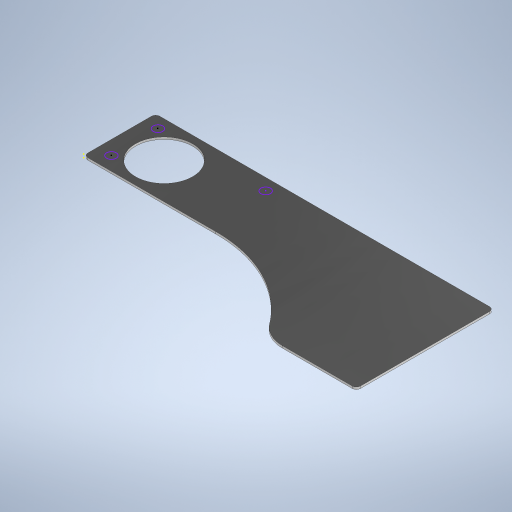
# Autodesk Inventor part: chapa_carbono_lateral_oposto
Saved by Autodesk Inventor 2024 (Build 280153000, 153)
## iProperties
Created: 2024-10-14
Part Number: chapa_carbono_lateral_oposto
Material: Genérico
Document SubType Name: Modeling
Designer: robof
Density: 1 g/cm^3
Appearance: Padrão
Author: robof
Autodesk Inventor part; units mm, degrees
ref_plane "YZ Plane" through (0, 0, 0) normal (1, 0, 0) x (0, 1, 0)
ref_plane "XZ Plane" through (0, 0, 0) normal (0, 1, 0) x (-1, 0, 0)
ref_plane "XY Plane" through (0, 0, 0) normal (0, 0, 1) x (1, 0, 0)
sketch "Esboço1" plane through (0, 0, 0) normal (0, 1, 0) x (-1, 0, 0)
  line L0 (0, 0) -> (-160, 0)
  line L1 (-160, 0) -> (-160, -34)
  line L2 (-160, -34) -> (0, -34)
  line L3 (0, -34) -> (0, 0)
  line L4 (0, 0) -> (-4, 0)
  line L5 (-4, 0) -> (-62.5, 0)
  line L6 (-160, -34) -> (-160, 31)
  line L7 (-160, -34) -> (-117, -34)
  line L8 (-117, -34) -> (-117, 31)
  line L9 (-117, 31) -> (-160, 31)
  line L10 (-160, 31) -> (-160, -34)
  arc A0 (-117, 31) -> (-62.5, 0) centre (-62.5, 63.4073) ccw
  dimension "d0" = 160
  dimension "d1" = 34
  dimension "d2" = 4
  dimension "d3" = 58.5
  dimension "d4" = 65
  dimension "d5" = 43
  constraints: 22 end point, 4 parallel, 3 point on line, 2 horizontal, 2 perpendicular, 2 point on circle, 1 centre point, 1 tangent
  measures "d0" distance of L2.end L1.end
  measures "d1" distance of L1.end L0.end
  measures "d2" distance of L0.start L4.end
  measures "d3" distance of L4.end L5.end
  measures "d4" distance of L1.end L6.end
  measures "d5" distance of L9.end L8.end
extrude "Extrusão1" add sketch "Esboço1" along normal blind 1
fillet "Arredondamento1" radius 2 4 edges at (160, 0.5, 31) (160, 0.5, -34) (0, 0.5, 0) (0, 0.5, -34)
fillet "Arredondamento2" radius 15 1 edges at (117, 0.5, 31)
sketch "Esboço5" plane through (0, 1, 0) normal (0, 1, 0) x (1, 0, 0)
  line L0 (160, -29) -> (160, 32) projected
  line L1 (160, -21.1735) -> (160, -7.1735)
  line L2 (160, -21.1735) -> (146, -21.1735)
  line L3 (124.952, -31) -> (158, -31) projected
  line L4 (146, -31) -> (139, -31)
  line L5 (146, -31) -> (146, -24)
  circle A0 centre (146, -24) radius 3.5
  line L6 (146, -24) -> (130, -24)
  circle A1 centre (130, -24) radius 3.5
  line L7 (146, -24) -> (146, 8)
  circle A2 centre (146, 8) radius 3.5
  line L8 (146, 8) -> (130, 8)
  circle A3 centre (130, 8) radius 3.5
  point P0 (0, 0)
  dimension "d32" = 14
  dimension "d33" = 14
  dimension "d34" = 7
  dimension "d35" = 7
  dimension "d36" = 7
  dimension "d37" = 16
  dimension "d38" = 7
  dimension "d39" = 32
  dimension "d40" = 7
  dimension "d41" = 7
  constraints: 14 end point, 4 centre point, 4 coincident, 4 point on line, 3 horizontal, 2 vertical
  measures "d32" distance of L1.start L1.end
  measures "d33" distance of L1.start L2.end
  measures "d34" distance of L4.start L4.end
  measures "d35" distance of L4.start L5.end
  measures "d36" diameter of A0
  measures "d37" distance of L6.start L6.end
  measures "d38" diameter of A1
  measures "d39" distance of L6.start L7.end
  measures "d40" diameter of A2
  measures "d41" diameter of A3
extrude "Extrusão3" add sketch "Esboço5" along normal blind 1
sketch "Esboço6" plane through (130, 2, -8) normal (0, 1, 0) x (1, 0, 0)
  circle A0 centre (0, 0) radius 2.25
  circle A1 centre (16, 0) radius 3.5 projected
  circle A2 centre (16, 0) radius 2.25
  circle A3 centre (0, -32) radius 3.5 projected
  circle A4 centre (0, -32) radius 2.25
  circle A5 centre (16, -32) radius 3.5 projected
  circle A6 centre (16, -32) radius 2.25
  point P0 (-130, -8)
  dimension "d44" = 4.5
  dimension "d45" = 4.5
  dimension "d46" = 4.5
  dimension "d47" = 4.5
  constraints: 4 centre point, 3 coincident
  measures "d44" diameter of A0
  measures "d45" diameter of A2
  measures "d46" diameter of A4
  measures "d47" diameter of A6
extrude "Extrusão4" add sketch "Esboço6" along normal blind 2.5 contours A0 | A2 | A4 | A6
sketch "Esboço7" plane through (130, 4.5, -8) normal (0, 1, 0) x (1, 0, 0)
  circle A0 centre (0, 0) radius 2.25 projected
  line L0 (-0.7066, -1.2286) -> (-1.4173, -0.0023)
  line L1 (-1.4173, -0.0023) -> (-0.7107, 1.2262)
  line L2 (-0.7107, 1.2262) -> (0.7066, 1.2286)
  line L3 (0.7066, 1.2286) -> (1.4173, 0.0023)
  line L4 (1.4173, 0.0023) -> (0.7107, -1.2262)
  line L5 (0.7107, -1.2262) -> (-0.7066, -1.2286)
  line L6 (0, 0) -> (8, 0)
  line L7 (8, 0) -> (8, -3.5397)
  circle A1 centre (16, 0) radius 2.25
  line L8 (16.7066, -1.2286) -> (17.4173, -0.0023)
  line L9 (17.4173, -0.0023) -> (16.7107, 1.2262)
  line L10 (16.7107, 1.2262) -> (15.2934, 1.2286)
  line L11 (15.2934, 1.2286) -> (14.5827, 0.0023)
  line L12 (14.5827, 0.0023) -> (15.2893, -1.2262)
  line L13 (15.2893, -1.2262) -> (16.7066, -1.2286)
  line L14 (0, 0) -> (0, -16)
  line L15 (0, -16) -> (6.7888, -16)
  circle A2 centre (0, -32) radius 2.25
  line L16 (-0.7066, -30.7714) -> (-1.4173, -31.9977)
  line L17 (-1.4173, -31.9977) -> (-0.7107, -33.2262)
  line L18 (-0.7107, -33.2262) -> (0.7066, -33.2286)
  line L19 (0.7066, -33.2286) -> (1.4173, -32.0023)
  line L20 (1.4173, -32.0023) -> (0.7107, -30.7738)
  line L21 (0.7107, -30.7738) -> (-0.7066, -30.7714)
  circle A3 centre (16, -32) radius 2.25
  line L22 (16.7066, -30.7714) -> (17.4173, -31.9977)
  line L23 (17.4173, -31.9977) -> (16.7107, -33.2262)
  line L24 (16.7107, -33.2262) -> (15.2934, -33.2286)
  line L25 (15.2934, -33.2286) -> (14.5827, -32.0023)
  line L26 (14.5827, -32.0023) -> (15.2893, -30.7738)
  line L27 (15.2893, -30.7738) -> (16.7066, -30.7714)
  point P0 (-130, -8)
  dimension "d50" = 8
  dimension "d51" = 16
  constraints: 56 end point, 24 symmetric about line, 4 coincident, 3 centre point, 2 perpendicular, 1 horizontal, 1 vertical, 16 other
  measures "d50" distance of L6.start L6.end
  measures "d51" distance of L6.start L14.end
extrude "Extrusão5" cut sketch "Esboço7" against normal blind 1.5 contours L6 L14 L5 L0 L1 L2 L3 L4 | L4 L5 L14 L6 | L13 L12 L11 L10 L9 L8 | L21 L20 L19 L18 L17 L16 | L22 L23 L24 L25 L26 L27
sketch "Esboço8" plane through (0, 1, 0) normal (0, 1, 0) x (1, 0, 0)
  line L0 (0, 0) -> (6, 0)
  line L1 (2, 0) -> (62.5, 0) projected
  line L2 (6, 0) -> (-1.5, 0)
  line L3 (6, 0) -> (6, 7.5)
  circle A0 centre (6, 7.5) radius 2.25
  line L4 (0, 32) -> (0, 2) projected
  line L5 (0, 17) -> (13.7618, 17)
  circle A1 centre (6, 26.5) radius 2.25
  dimension "d54" = 6
  dimension "d55" = 7.5
  dimension "d56" = 7.5
  dimension "d57" = 4.5
  constraints: 8 end point, 2 centre point, 2 point on line, 1 coincident, 1 horizontal, 1 midpoint, 1 symmetric about line, 1 vertical, 1 other
  measures "d54" distance of L0.start L0.end
  measures "d55" distance of L0.end L2.end
  measures "d56" distance of L0.end L3.end
  measures "d57" diameter of A0
extrude "Extrusão6" cut sketch "Esboço8" against normal blind 0.1
sketch "Esboço9" plane through (6, 0.9, -26.5) normal (0, 1, 0) x (1, 0, 0)
  circle A0 centre (0, -19) radius 2.25 projected
  line L0 (0, -19) -> (0.25, -19)
  line L1 (0.25, -19) -> (0.25, -20.5)
  line L2 (0.25, -20.5) -> (0, -20.5)
  line L3 (0, -20.5) -> (0, -19)
  line L4 (0, -20.5) -> (-0.25, -20.5)
  line L5 (-0.25, -20.5) -> (-0.25, -19)
  line L6 (-0.25, -19) -> (0, -19)
  line L7 (0, -19) -> (0, -20.5)
  line L8 (0.25, -20.5) -> (-0.25, -20.5)
  line L9 (-0.25, -20.5) -> (-0.25, -17.5)
  line L10 (-0.25, -17.5) -> (0.25, -17.5)
  line L11 (0.25, -17.5) -> (0.25, -20.5)
  line L12 (0, -19) -> (1.5, -19)
  line L13 (1.5, -19) -> (1.5, -18.75)
  line L14 (1.5, -18.75) -> (0, -18.75)
  line L15 (0, -18.75) -> (0, -19)
  line L16 (1.5, -18.75) -> (-1.5, -18.75)
  line L17 (-1.5, -18.75) -> (-1.5, -19.25)
  line L18 (-1.5, -19.25) -> (1.5, -19.25)
  line L19 (1.5, -19.25) -> (1.5, -18.75)
  line L20 (-6, 5.5) -> (-6, -24.5) projected
  line L21 (-6, -9.5) -> (4.7143, -9.5)
  line L22 (0, 0) -> (0.25, 0)
  line L23 (0.25, 0) -> (0.25, 1.5)
  line L24 (0.25, 1.5) -> (0, 1.5)
  line L25 (0, 1.5) -> (0, 0)
  line L26 (0, 1.5) -> (-0.25, 1.5)
  line L27 (-0.25, 1.5) -> (-0.25, 0)
  line L28 (-0.25, 0) -> (0, 0)
  line L29 (0, 0) -> (0, 1.5)
  line L30 (0.25, 1.5) -> (-0.25, 1.5)
  line L31 (-0.25, 1.5) -> (-0.25, -1.5)
  line L32 (-0.25, -1.5) -> (0.25, -1.5)
  line L33 (0.25, -1.5) -> (0.25, 1.5)
  line L34 (0, 0) -> (1.5, 0)
  line L35 (1.5, 0) -> (1.5, -0.25)
  line L36 (1.5, -0.25) -> (0, -0.25)
  line L37 (0, -0.25) -> (0, 0)
  line L38 (1.5, -0.25) -> (-1.5, -0.25)
  line L39 (-1.5, -0.25) -> (-1.5, 0.25)
  line L40 (-1.5, 0.25) -> (1.5, 0.25)
  line L41 (1.5, 0.25) -> (1.5, -0.25)
  point P0 (-6, -26.5)
  point P1 (-0.25, -19.25)
  point P2 (0.25, -19.25)
  point P3 (0.25, -18.75)
  point P4 (-0.25, -18.75)
  point P5 (0.25, 0.25)
  point P6 (-0.25, 0.25)
  point P7 (-0.25, -0.25)
  point P8 (0.25, -0.25)
  dimension "d60" = 0.25
  dimension "d61" = 1.5
  dimension "d62" = 0.25
  dimension "d63" = 3
  dimension "d64" = 1.5
  dimension "d65" = 0.25
  dimension "d66" = 3
  dimension "d67" = 0.5
  constraints: 82 end point, 16 symmetric about line, 10 parallel, 6 horizontal, 5 perpendicular, 4 point on line, 1 midpoint
  measures "d60" distance of L1.end L2.end
  measures "d61" distance of L0.end L1.end
  measures "d62" distance of L5.end L6.end
  measures "d63" distance of L8.end L9.end
  measures "d64" distance of L14.end L13.end
  measures "d65" distance of L13.end L12.end
  measures "d66" distance of L18.end L17.end
  measures "d67" distance of L17.end L16.end
extrude "Extrusão7" cut sketch "Esboço9" against normal blind 0.1 contours L15 L14 L11 L0 | L0 L1 L18 L3 | L3 L18 L5 L6 | L6 L9 L16 L15 | L12 L19 L18 L1 | L11 L14 L13 L12 | L18 L1 L2 L3 | L3 L4 L5 L18 | L5 L18 L17 L16 L9 | L16 L9 L10 L11 L14 | L25 L40 L23 L22 | L28 L27 L40 L25 | L37 L38 L31 L28 | L22 L33 L36 L37 | L34 L35 L36 L33 | L23 L40 L41 L34 | L40 L27 L26 L25 | L25 L24 L23 L40 | L31 L38 L39 L40 L27 | L36 L33 L32 L31 L38
sketch "Esboço10" plane through (6, 0.9, -26.5) normal (0, 1, 0) x (1, 0, 0)
  line L0 (0, 0) -> (52, 0)
  circle A0 centre (52, 0) radius 2.25
  circle A1 centre (0, -19) radius 2.25 projected
  line L1 (0, -19) -> (52, -19)
  circle A2 centre (52, -19) radius 2.25
  point P0 (-6, -26.5)
  dimension "d70" = 52
  dimension "d71" = 4.5
  dimension "d72" = 52
  dimension "d73" = 4.5
  constraints: 4 end point, 2 centre point, 2 coincident, 1 horizontal, 1 parallel
  measures "d70" distance of L0.start L0.end
  measures "d71" diameter of A0
  measures "d72" distance of L1.start L1.end
  measures "d73" diameter of A2
extrude "Extrusão8" cut sketch "Esboço10" along normal blind 2 contours A0 | A2
sketch "Esboço11" plane through (58, 0.9, -26.5) normal (0, 1, 0) x (1, 0, 0)
  line L0 (0, 0) -> (0.25, 0)
  line L1 (0.25, 0) -> (0.25, 1.5)
  line L2 (0.25, 1.5) -> (0, 1.5)
  line L3 (0, 1.5) -> (0, 0)
  line L4 (0.25, 1.5) -> (-0.25, 1.5)
  line L5 (-0.25, 1.5) -> (-0.25, -1.5)
  line L6 (-0.25, -1.5) -> (0.25, -1.5)
  line L7 (0.25, -1.5) -> (0.25, 1.5)
  line L8 (0, 0) -> (1.5, 0)
  line L9 (1.5, 0) -> (1.5, 0.25)
  line L10 (1.5, 0.25) -> (0, 0.25)
  line L11 (0, 0.25) -> (0, 0)
  line L12 (1.5, 0.25) -> (-1.5, 0.25)
  line L13 (-1.5, 0.25) -> (-1.5, -0.25)
  line L14 (-1.5, -0.25) -> (1.5, -0.25)
  line L15 (1.5, -0.25) -> (1.5, 0.25)
  line L16 (-58, 5.5) -> (-58, -24.5) projected
  line L17 (-58, -9.5) -> (-46.2393, -9.5)
  line L18 (0, -19) -> (0.25, -19)
  line L19 (0.25, -19) -> (0.25, -20.5)
  line L20 (0.25, -20.5) -> (0, -20.5)
  line L21 (0, -20.5) -> (0, -19)
  line L22 (0.25, -20.5) -> (-0.25, -20.5)
  line L23 (-0.25, -20.5) -> (-0.25, -17.5)
  line L24 (-0.25, -17.5) -> (0.25, -17.5)
  line L25 (0.25, -17.5) -> (0.25, -20.5)
  line L26 (0, -19) -> (1.5, -19)
  line L27 (1.5, -19) -> (1.5, -19.25)
  line L28 (1.5, -19.25) -> (0, -19.25)
  line L29 (0, -19.25) -> (0, -19)
  line L30 (1.5, -19.25) -> (-1.5, -19.25)
  line L31 (-1.5, -19.25) -> (-1.5, -18.75)
  line L32 (-1.5, -18.75) -> (1.5, -18.75)
  line L33 (1.5, -18.75) -> (1.5, -19.25)
  point P0 (-58, -26.5)
  point P1 (0.25, -0.25)
  point P2 (1.5, 0)
  point P3 (0.25, 0.25)
  point P4 (0, 1.5)
  point P5 (-0.25, 0.25)
  point P6 (-0.25, -0.25)
  point P7 (0.25, -19.25)
  point P8 (1.5, -19)
  point P9 (0.25, -18.75)
  point P10 (-0.25, -18.75)
  point P11 (-0.25, -19.25)
  dimension "d76" = 0.25
  dimension "d77" = 1.5
  dimension "d78" = 0.5
  dimension "d79" = 3
  dimension "d80" = 1.5
  dimension "d81" = 0.25
  dimension "d82" = 3
  dimension "d83" = 0.5
  constraints: 66 end point, 13 symmetric about line, 8 parallel, 5 horizontal, 4 perpendicular, 1 midpoint
  measures "d76" distance of L2.end L1.end
  measures "d77" distance of L1.end L0.end
  measures "d78" distance of L6.end L5.end
  measures "d79" distance of L5.end L4.end
  measures "d80" distance of L10.end L9.end
  measures "d81" distance of L9.end L8.end
  measures "d82" distance of L14.end L13.end
  measures "d83" distance of L13.end L12.end
extrude "Extrusão9" cut sketch "Esboço11" against normal blind 0.1
sketch "Esboço12" plane through (0, 1, 0) normal (0, 1, 0) x (1, 0, 0)
  line L0 (0, 32) -> (0, 2) projected
  line L1 (0, 17) -> (5, 17)
  line L2 (5, 17) -> (36, 17)
  line L3 (5, 17) -> (20.5, 17)
  circle A0 centre (20.5, 17) radius 13
  point P0 (0, 0)
  dimension "d86" = 5
  dimension "d87" = 31
  dimension "d88" = 15.5
  dimension "d89" = 26
  constraints: 6 end point, 2 midpoint, 1 centre point, 1 coincident, 1 horizontal, 1 point on line
  measures "d86" distance of L1.start L1.end
  measures "d87" distance of L1.end L2.end
  measures "d88" distance of L1.end L3.end
  measures "d89" diameter of A0
extrude "Extrusão10" cut sketch "Esboço12" against normal blind 10
sketch "Esboço13" plane through (0, 1, 0) normal (0, 1, 0) x (1, 0, 0)
  circle A0 centre (20.5, 17) radius 13 projected
  circle A1 centre (20.5, 17) radius 13
  point P0 (0, 0)
  constraints: 1 centre point, 1 coincident
extrude "Extrusão11" add sketch "Esboço13" against normal blind 1
sketch "Esboço14" plane through (0, 1, 0) normal (0, 1, 0) x (1, 0, 0)
  line L0 (0, 32) -> (0, 2) projected
  line L1 (0, 17) -> (4.15, 17)
  line L2 (4.15, 17) -> (15.55, 17)
  line L3 (16.6408, 0) -> (16.6408, 6)
  circle A0 centre (15.55, 17) radius 11.054
  circle A1 centre (6, 7.5) radius 2.25 projected
  circle A2 centre (6, 7.5) radius 2.25
  circle A3 centre (6, 26.5) radius 2.25 projected
  circle A4 centre (6, 26.5) radius 2.25
  point P0 (0, 0)
  dimension "d94" = 4.15
  dimension "d95" = 11.4
  dimension "d97" = 6
  constraints: 6 end point, 3 coincident, 2 centre point, 2 horizontal, 1 midpoint, 1 vertical, 3 other
  measures "d94" distance of L1.start L1.end
  measures "d95" distance of L1.end L2.end
  measures "d97" distance of L3.start L3.end
extrude "Extrusão12" add sketch "Esboço14" against normal blind 1 contours A1 | A3
sketch "Esboço15" plane through (0, 1, 0) normal (0, 1, 0) x (1, 0, 0)
  circle A0 centre (58, 7.5) radius 2.25 projected
  circle A1 centre (58, 7.5) radius 2.25
  circle A2 centre (58, 26.5) radius 2.25 projected
  circle A3 centre (58, 26.5) radius 2.25
  point P0 (0, 0)
  constraints: 2 centre point, 2 coincident
extrude "Extrusão13" add sketch "Esboço15" against normal blind 1
sketch "Esboço16" plane through (0, 1, 0) normal (0, 1, 0) x (1, 0, 0)
  line L0 (0, 0) -> (7, 0)
  line L1 (7, 0) -> (7, 6)
  line L2 (7, 6) -> (0, 6)
  line L3 (0, 6) -> (0, 0)
  circle A0 centre (7, 6) radius 2.25
  line L4 (0, 32) -> (0, 2) projected
  line L5 (0, 17) -> (5.9961, 17)
  line L6 (7, 0) -> (32.5, 0)
  line L7 (2, 0) -> (62.5, 0) projected
  line L8 (32.5, 0) -> (32.5, 15.1049)
  circle A1 centre (7, 28) radius 2.25
  circle A2 centre (58, 6) radius 2.25
  circle A3 centre (58, 28) radius 2.25
  dimension "d102" = 7
  dimension "d103" = 6
  dimension "d104" = 4.5
  dimension "d105" = 25.5
  constraints: 14 end point, 4 centre point, 3 symmetric about line, 2 horizontal, 2 parallel, 1 coincident, 1 midpoint, 1 perpendicular, 1 point on line, 1 vertical, 3 other
  measures "d102" distance of L2.end L1.end
  measures "d103" distance of L1.end L0.end
  measures "d104" diameter of A0
  measures "d105" distance of L0.end L6.end
extrude "Extrusão14" cut sketch "Esboço16" against normal blind 1 contours A0 L2 L1 | L1 L2 A0 | A1 | A2 | A3
sketch "Esboço17" plane through (0, 1, 0) normal (0, 1, 0) x (1, 0, 0)
  line L0 (0, 32) -> (0, 2) projected
  line L1 (0, 17) -> (17, 17)
  line L2 (17, 17) -> (21, 17)
  circle A0 centre (21, 17) radius 13.5
  point P0 (0, 0)
  dimension "d108" = 17
  dimension "d109" = 4
  dimension "d110" = 27
  constraints: 4 end point, 2 horizontal, 1 centre point, 1 coincident, 1 midpoint
  measures "d108" distance of L1.start L1.end
  measures "d109" distance of L1.end L2.end
  measures "d110" diameter of A0
extrude "Extrusão15" cut sketch "Esboço17" against normal blind 1
sketch "Esboço18" plane through (0, 0, 0) normal (0, -1, 0) x (1, 0, 0)
  circle A0 centre (58, -6) radius 2.25 projected
  circle A1 centre (58, -6) radius 2.25
  circle A2 centre (58, -28) radius 2.25 projected
  circle A3 centre (58, -28) radius 2.25
  circle A4 centre (7, -28) radius 2.25 projected
  circle A5 centre (7, -28) radius 2.25
  circle A6 centre (7, -6) radius 2.25 projected
  circle A7 centre (7, -6) radius 2.25
  point P0 (0, 0)
  constraints: 4 centre point, 4 coincident
extrude "Extrusão16" add sketch "Esboço18" against normal blind 2
sketch "Esboço19" plane through (7, 2, -28) normal (0, 1, 0) x (1, 0, 0)
  circle A0 centre (0, 0) radius 2.25
  circle A1 centre (0, -22) radius 2.25 projected
  circle A2 centre (0, -22) radius 2.25
  circle A3 centre (51, 0) radius 2.25 projected
  circle A4 centre (51, 0) radius 2.25
  circle A5 centre (51, -22) radius 2.25 projected
  circle A6 centre (51, -22) radius 2.25
  point P0 (-7, -28)
  constraints: 4 centre point, 3 coincident
extrude "Extrusão17" cut sketch "Esboço19" against normal blind 0.5
sketch "Esboço20" plane through (7, 1.5, -28) normal (0, 1, 0) x (1, 0, 0)
  line L0 (0, 0) -> (0.3, 0)
  line L1 (0.3, 0) -> (0.3, 1.6)
  line L2 (0.3, 1.6) -> (0, 1.6)
  line L3 (0, 1.6) -> (0, 0)
  line L4 (0.3, 0) -> (-0.3, 0)
  line L5 (-0.3, 0) -> (-0.3, 1.6)
  line L6 (-0.3, 1.6) -> (0.3, 1.6)
  line L7 (0.3, 1.6) -> (0.3, 0)
  line L8 (-0.9434, 0) -> (0.9565, 0)
  line L9 (0.3, 0) -> (0.3, -1.6)
  line L10 (-0.3, 0) -> (-0.3, -1.6)
  line L11 (-0.3, -1.6) -> (0.3, -1.6)
  line L12 (-0.3, 0) -> (-0.3, 0.3)
  line L13 (-0.3, 0.3) -> (-1.9, 0.3)
  line L14 (-1.9, 0.3) -> (-1.9, -0.3)
  line L15 (-1.9, -0.3) -> (-0.3, -0.3)
  line L16 (-0.3, -0.3) -> (-0.3, 0.3)
  line L17 (0.3, 0.3) -> (1.9, 0.3)
  line L18 (1.9, 0.3) -> (1.9, -0.3)
  line L19 (1.9, -0.3) -> (0.3, -0.3)
  line L20 (-1.9, -0.3) -> (-1.6, -0.3)
  line L21 (-1.6, -0.3) -> (-1.6, 0.3)
  line L22 (1.6, -0.3) -> (1.6, 0.3)
  line L23 (-7, 4) -> (-7, -26) projected
  line L24 (-7, -11) -> (4.0059, -11)
  line L25 (151, 6) -> (-5, 6) projected
  line L26 (0, 6) -> (25.5, 6)
  line L27 (25.5, 6) -> (25.5, -11)
  line L28 (0.3, -22) -> (0.3, -23.6)
  line L29 (-0.3, -22) -> (-0.3, -23.6)
  line L30 (-0.3, -23.6) -> (0.3, -23.6)
  line L31 (-0.3, -22) -> (-0.3, -20.4)
  line L32 (-0.3, -20.4) -> (0.3, -20.4)
  line L33 (0.3, -22) -> (0.3, -20.4)
  line L34 (-0.3, -22.3) -> (-1.9, -22.3)
  line L35 (-1.9, -21.7) -> (-0.3, -21.7)
  line L36 (0.3, -22.3) -> (1.9, -22.3)
  line L37 (1.9, -21.7) -> (0.3, -21.7)
  line L38 (-1.6, -21.7) -> (-1.6, -22.3)
  line L39 (1.6, -21.7) -> (1.6, -22.3)
  line L40 (51, 0) -> (50.7, 0)
  line L41 (50.7, 0) -> (50.7, 1.6)
  line L42 (50.7, 1.6) -> (51, 1.6)
  line L43 (51, 1.6) -> (51, 0)
  line L44 (50.7, 0) -> (51.3, 0)
  line L45 (51.3, 0) -> (51.3, 1.6)
  line L46 (51.3, 1.6) -> (50.7, 1.6)
  line L47 (50.7, 1.6) -> (50.7, 0)
  line L48 (51.9434, 0) -> (50.0435, 0)
  line L49 (51.3, 0) -> (51.3, -1.6)
  line L50 (51.3, -1.6) -> (50.7, -1.6)
  line L51 (50.7, 0) -> (50.7, -1.6)
  line L52 (51.3, 0) -> (51.3, 0.3)
  line L53 (51.3, 0.3) -> (52.9, 0.3)
  line L54 (52.9, 0.3) -> (52.9, -0.3)
  line L55 (52.9, -0.3) -> (51.3, -0.3)
  line L56 (51.3, -0.3) -> (51.3, 0.3)
  line L57 (50.7, 0.3) -> (49.1, 0.3)
  line L58 (49.1, 0.3) -> (49.1, -0.3)
  line L59 (49.1, -0.3) -> (50.7, -0.3)
  line L60 (52.9, -0.3) -> (52.6, -0.3)
  line L61 (52.6, -0.3) -> (52.6, 0.3)
  line L62 (49.4, -0.3) -> (49.4, 0.3)
  line L63 (51.3, -23.6) -> (50.7, -23.6)
  line L64 (51.3, -22) -> (51.3, -23.6)
  line L65 (50.7, -22) -> (50.7, -23.6)
  line L66 (50.7, -22.3) -> (49.1, -22.3)
  line L67 (49.4, -21.7) -> (49.4, -22.3)
  line L68 (49.1, -21.7) -> (50.7, -21.7)
  line L69 (50.7, -22) -> (50.7, -20.4)
  line L70 (51.3, -22) -> (51.3, -20.4)
  line L71 (52.9, -21.7) -> (51.3, -21.7)
  line L72 (52.6, -21.7) -> (52.6, -22.3)
  line L73 (51.3, -22.3) -> (52.9, -22.3)
  line L74 (51.3, -20.4) -> (50.7, -20.4)
  point P0 (-7, -28)
  point P1 (46.9941, -11)
  point P2 (0.3, -23.6)
  point P3 (0.3, -22.3)
  point P4 (0.3, -21.7)
  point P5 (0.3, -20.4)
  point P6 (-0.3, -21.7)
  point P7 (0.3, 0.3)
  point P8 (0, 1.6)
  point P9 (-0.3, -0.3)
  point P10 (0.3, -1.6)
  point P11 (0.3, -0.3)
  point P12 (1.6, -0.3)
  point P13 (1.6, 0.3)
  point P14 (50.7, -0.3)
  point P15 (50.7, -1.6)
  point P16 (51.3, -0.3)
  point P17 (51, 1.6)
  point P18 (50.7, 0.3)
  point P19 (49.4, 0.3)
  point P20 (49.4, -0.3)
  dimension "d117" = 0.3
  dimension "d118" = 1.6
  dimension "d119" = 0.6
  dimension "d120" = 1.6
  dimension "d121" = 0.3
  dimension "d122" = 1.6
  dimension "d123" = 0.6
  dimension "d124" = 0.3
  dimension "d125" = 25.5
  constraints: 146 end point, 74 symmetric about line, 18 point on line, 6 parallel, 5 perpendicular, 4 horizontal, 1 midpoint
  measures "d117" distance of L2.end L1.end
  measures "d118" distance of L1.end L0.end
  measures "d119" distance of L5.end L6.end
  measures "d120" distance of L4.end L5.end
  measures "d121" distance of L4.end L12.end
  measures "d122" distance of L15.end L14.end
  measures "d123" distance of L14.end L13.end
  measures "d124" distance of L14.end L20.end
  measures "d125" distance of L26.start L26.end
extrude "Extrusão18" cut sketch "Esboço20" against normal blind 0.5 contours L3 L2 L1 L0 | L4 L5 L6 L3 | L0 L9 L11 L10 L4 | L1 L17 L22 L19 L9 | L10 L15 L21 L13 L5 | L33 L37 L39 L36 L28 | L28 L30 L29 L31 L32 L33 | L34 L38 L35 L31 L29 | L44 L49 L50 L51 L40 | L40 L41 L42 L43 | L43 L46 L45 L44 | L51 L59 L62 L57 L41 | L45 L53 L61 L55 L49 | L63 L65 L69 L74 L70 L64 | L64 L70 L71 L72 L73 | L66 L67 L68 L69 L65
sketch "Esboço21" plane through (0, 0, 0) normal (0, -1, 0) x (1, 0, 0)
  point P0 (0, 0)
sketch "Esboço22" plane through (0, 0, 0) normal (0, -1, 0) x (1, 0, 0)
  circle A0 centre (130, -8) radius 2.25 projected
  circle A1 centre (130, -8) radius 3.5
  circle A2 centre (146, -8) radius 3.5 projected
  circle A3 centre (146, -8) radius 3.5
  circle A4 centre (130, 24) radius 3.5 projected
  circle A5 centre (130, 24) radius 3.5
  circle A6 centre (146, 24) radius 3.5 projected
  circle A7 centre (146, 24) radius 3.5
  point P0 (0, 0)
  constraints: 4 centre point, 4 coincident
extrude "Extrusão19" add sketch "Esboço22" along normal blind 1 contours A0 | A1 | A2 | A4 | A6
sketch "Esboço23" plane through (130, 4.5, -8) normal (0, 1, 0) x (1, 0, 0)
  circle A0 centre (0, 0) radius 3.5 projected
  circle A1 centre (0, 0) radius 3.5
  circle A2 centre (16, 0) radius 2.25 projected
  circle A3 centre (16, 0) radius 3.5
  circle A4 centre (0, -32) radius 2.25 projected
  circle A5 centre (0, -32) radius 3.5
  circle A6 centre (16, -32) radius 2.25 projected
  circle A7 centre (16, -32) radius 3.5
  point P0 (-130, -8)
  constraints: 4 centre point, 4 coincident
extrude "Extrusão20" cut sketch "Esboço23" against normal blind 3.5 contours A0 | A2 | A3 | A4 | A5 | A6 | A7
sketch "Esboço24" plane through (58, 1.5, -6) normal (0, 1, 0) x (1, 0, 0)
  circle A0 centre (-51, 0) radius 2.25 projected
  circle A1 centre (-51, 0) radius 2.25
  circle A2 centre (-51, 22) radius 2.25 projected
  circle A3 centre (-51, 22) radius 2.25
  circle A4 centre (-0.0001, 22) radius 2.2501
  circle A5 centre (-51, 0) radius 2.25
  point P0 (-58, -6)
  constraints: 4 centre point, 3 coincident, 1 concentric
sketch "Esboço25" plane through (0, 0, 0) normal (0, -1, 0) x (1, 0, 0)
  circle A0 centre (7, -28) radius 2.25 projected
  circle A1 centre (7, -28) radius 2.25
  circle A2 centre (7, -6) radius 2.25 projected
  circle A3 centre (7, -6) radius 2.25
  circle A4 centre (58, -6) radius 2.25 projected
  circle A5 centre (58, -6) radius 2.25
  circle A6 centre (58, -28) radius 2.25 projected
  circle A7 centre (58, -28) radius 2.25
  point P0 (0, 0)
  constraints: 4 centre point, 4 coincident
extrude "Extrusão21" cut sketch "Esboço25" against normal blind 0.5
sketch "Esboço26" plane through (7, 0.5, -6) normal (0, -1, 0) x (1, 0, 0)
  line L0 (0.3, 0.3) -> (0.3, 1.6) projected
  line L1 (0.3, 0.3) -> (0.3, 1.6)
  line L2 (-0.3, 1.6) -> (-0.3, 0.3) projected
  line L3 (0.3, 1.6) -> (-0.3, 1.6)
  line L4 (-0.3, 0.3) -> (-1.6, 0.3) projected
  line L5 (-0.3, 1.6) -> (-0.3, 0.3)
  line L6 (-0.3, 0.3) -> (-1.6, 0.3)
  line L7 (-1.6, 0.3) -> (-1.6, -0.3) projected
  line L8 (-1.6, 0.3) -> (-1.6, -0.3)
  line L9 (-0.3, -0.3) -> (-0.3, -1.6) projected
  line L10 (-1.6, -0.3) -> (-0.3, -0.3)
  line L11 (-0.3, -0.3) -> (-0.3, -1.6)
  line L12 (-0.3, -1.6) -> (0.3, -1.6)
  line L13 (0.3, -1.6) -> (0.3, -0.3)
  line L14 (1.6, -0.3) -> (1.6, 0.3) projected
  line L15 (0.3, -0.3) -> (1.6, -0.3)
  line L16 (1.6, -0.3) -> (1.6, 0.3)
  line L17 (1.6, 0.3) -> (0.3, 0.3) projected
  line L18 (1.6, 0.3) -> (0.3, 0.3)
  line L19 (-7, -26) -> (-7, 4) projected
  line L20 (-7, -11) -> (-0.6062, -11)
  line L21 (0, 0) -> (25.5, 0)
  line L22 (25.5, 0) -> (25.5, 6)
  line L23 (-5, 6) -> (55.5, 6) projected
  line L24 (0.3, -22.3) -> (0.3, -23.6)
  line L25 (0.3, -22.3) -> (0.3, -23.6)
  line L26 (-0.3, -23.6) -> (-0.3, -22.3)
  line L27 (0.3, -23.6) -> (-0.3, -23.6)
  line L28 (-0.3, -22.3) -> (-1.6, -22.3)
  line L29 (-0.3, -23.6) -> (-0.3, -22.3)
  line L30 (-0.3, -22.3) -> (-1.6, -22.3)
  line L31 (-1.6, -22.3) -> (-1.6, -21.7)
  line L32 (-1.6, -22.3) -> (-1.6, -21.7)
  line L33 (-0.3, -21.7) -> (-0.3, -20.4)
  line L34 (-1.6, -21.7) -> (-0.3, -21.7)
  line L35 (-0.3, -21.7) -> (-0.3, -20.4)
  line L36 (-0.3, -20.4) -> (0.3, -20.4)
  line L37 (0.3, -20.4) -> (0.3, -21.7)
  line L38 (1.6, -21.7) -> (1.6, -22.3)
  line L39 (0.3, -21.7) -> (1.6, -21.7)
  line L40 (1.6, -21.7) -> (1.6, -22.3)
  line L41 (1.6, -22.3) -> (0.3, -22.3)
  line L42 (1.6, -22.3) -> (0.3, -22.3)
  line L43 (50.7, 0.3) -> (50.7, 1.6)
  line L44 (50.7, 0.3) -> (50.7, 1.6)
  line L45 (51.3, 1.6) -> (51.3, 0.3)
  line L46 (50.7, 1.6) -> (51.3, 1.6)
  line L47 (51.3, 0.3) -> (52.6, 0.3)
  line L48 (51.3, 1.6) -> (51.3, 0.3)
  line L49 (51.3, 0.3) -> (52.6, 0.3)
  line L50 (52.6, 0.3) -> (52.6, -0.3)
  line L51 (52.6, 0.3) -> (52.6, -0.3)
  line L52 (51.3, -0.3) -> (51.3, -1.6)
  line L53 (52.6, -0.3) -> (51.3, -0.3)
  line L54 (51.3, -0.3) -> (51.3, -1.6)
  line L55 (51.3, -1.6) -> (50.7, -1.6)
  line L56 (50.7, -1.6) -> (50.7, -0.3)
  line L57 (49.4, -0.3) -> (49.4, 0.3)
  line L58 (50.7, -0.3) -> (49.4, -0.3)
  line L59 (49.4, -0.3) -> (49.4, 0.3)
  line L60 (49.4, 0.3) -> (50.7, 0.3)
  line L61 (49.4, 0.3) -> (50.7, 0.3)
  line L62 (50.7, -22.3) -> (50.7, -23.6)
  line L63 (50.7, -22.3) -> (50.7, -23.6)
  line L64 (51.3, -23.6) -> (51.3, -22.3)
  line L65 (50.7, -23.6) -> (51.3, -23.6)
  line L66 (51.3, -22.3) -> (52.6, -22.3)
  line L67 (51.3, -23.6) -> (51.3, -22.3)
  line L68 (51.3, -22.3) -> (52.6, -22.3)
  line L69 (49.4, -21.7) -> (49.4, -22.3)
  line L70 (50.7, -21.7) -> (49.4, -21.7)
  line L71 (49.4, -21.7) -> (49.4, -22.3)
  line L72 (49.4, -22.3) -> (50.7, -22.3)
  line L73 (49.4, -22.3) -> (50.7, -22.3)
  line L74 (52.6, -22.3) -> (52.6, -21.7)
  line L75 (52.6, -21.7) -> (51.3, -21.7)
  line L76 (51.3, -20.4) -> (50.7, -20.4)
  line L77 (50.7, -20.4) -> (50.7, -21.7)
  line L78 (51.3, -21.7) -> (51.3, -20.4)
  line L79 (51.3, -21.7) -> (51.3, -20.4)
  line L80 (52.6, -22.3) -> (52.6, -21.7)
  point P0 (-7, 6)
  point P1 (0, -22)
  point P2 (51.6062, -11)
  point P3 (51, 0)
  point P4 (51, -22)
  dimension "d134" = 25.5
  constraints: 144 end point, 40 symmetric about line, 13 point on line, 8 perpendicular, 4 collinear, 2 horizontal, 1 midpoint
  measures "d134" distance of L21.start L21.end
extrude "Extrusão22" add sketch "Esboço26" along normal blind 0.5
sketch "Esboço27" plane through (130, -1, -8) normal (0, -1, 0) x (1, 0, 0)
  circle A0 centre (0, 0) radius 2.25
  circle A1 centre (16, 0) radius 3.5 projected
  circle A2 centre (16, 0) radius 2.25
  circle A3 centre (16, 32) radius 3.5 projected
  circle A4 centre (16, 32) radius 2.25
  circle A5 centre (0, 32) radius 3.5 projected
  circle A6 centre (0, 32) radius 2.25
  point P0 (-130, 8)
  dimension "d137" = 4.5
  dimension "d138" = 4.5
  dimension "d139" = 4.5
  dimension "d140" = 4.5
  constraints: 4 centre point, 3 coincident
  measures "d137" diameter of A0
  measures "d138" diameter of A2
  measures "d139" diameter of A4
  measures "d140" diameter of A6
extrude "Extrusão23" add sketch "Esboço27" along normal blind 2.5 contours A0 | A2 | A4 | A6
sketch "Esboço28" plane through (130, -3.5, 24) normal (0, -1, 0) x (1, 0, 0)
  circle A0 centre (0, 0) radius 2.25 projected
  line L0 (0, -1.4971) -> (-1.2965, -0.7485)
  line L1 (-1.2965, -0.7485) -> (-1.2965, 0.7485)
  line L2 (-1.2965, 0.7485) -> (0, 1.4971)
  line L3 (0, 1.4971) -> (1.2965, 0.7485)
  line L4 (1.2965, 0.7485) -> (1.2965, -0.7485)
  line L5 (1.2965, -0.7485) -> (0, -1.4971)
  line L6 (0, 0) -> (8, 0)
  line L7 (8, 0) -> (8, 7)
  line L8 (-5.048, 7) -> (28, 7) projected
  circle A1 centre (16, 0) radius 2.25 projected
  line L9 (16, 0) -> (16, -16)
  line L10 (16, -16) -> (30, -16)
  line L11 (30, 5) -> (30, -56) projected
  line L12 (16, -1.4971) -> (17.2965, -0.7485)
  line L13 (17.2965, -0.7485) -> (17.2965, 0.7485)
  line L14 (17.2965, 0.7485) -> (16, 1.4971)
  line L15 (16, 1.4971) -> (14.7035, 0.7485)
  line L16 (14.7035, 0.7485) -> (14.7035, -0.7485)
  line L17 (14.7035, -0.7485) -> (16, -1.4971)
  line L18 (0, -30.5029) -> (-1.2965, -31.2515)
  line L19 (-1.2965, -31.2515) -> (-1.2965, -32.7485)
  line L20 (-1.2965, -32.7485) -> (0, -33.4971)
  line L21 (0, -33.4971) -> (1.2965, -32.7485)
  line L22 (1.2965, -32.7485) -> (1.2965, -31.2515)
  line L23 (1.2965, -31.2515) -> (0, -30.5029)
  line L24 (17.2965, -32.7485) -> (16, -33.4971)
  line L25 (16, -33.4971) -> (14.7035, -32.7485)
  line L26 (14.7035, -32.7485) -> (14.7035, -31.2515)
  line L27 (14.7035, -31.2515) -> (16, -30.5029)
  line L28 (16, -30.5029) -> (17.2965, -31.2515)
  line L29 (17.2965, -31.2515) -> (17.2965, -32.7485)
  point P0 (-130, -24)
  dimension "d143" = 8
  dimension "d144" = 16
  constraints: 56 end point, 18 symmetric about line, 2 perpendicular, 2 point on line, 1 coincident, 1 horizontal, 1 parallel, 13 other
  measures "d143" distance of L6.start L6.end
  measures "d144" distance of L9.start L9.end
extrude "Extrusão24" cut sketch "Esboço28" against normal blind 1.5 contours L0 L1 L2 L3 L4 L5 | L17 L16 L15 L14 L13 L12 | L23 L22 L21 L20 L19 L18 | L24 L25 L26 L27 L28 L29
sketch "Esboço29" plane through (58, 1.5, -6) normal (0, 1, 0) x (1, 0, 0)
  circle A0 centre (0, 0) radius 2.25 projected
  circle A1 centre (0, 0) radius 2.25
  circle A2 centre (0, 0) radius 2.25 projected
  circle A3 centre (0, 0) radius 2.25
  line L0 (-55.513, -3.9178) -> (4.5882, -3.9178)
  line L1 (4.5882, -3.9178) -> (4.5882, 26.4667)
  line L2 (4.5882, 26.4667) -> (-55.513, 26.4667)
  line L3 (-55.513, 26.4667) -> (-55.513, -3.9178)
  point P0 (-58, -6)
  constraints: 8 end point, 2 centre point, 2 coincident, 2 parallel, 1 concentric, 1 horizontal, 1 perpendicular
extrude "Extrusão25" cut sketch "Esboço29" against normal blind 0.5
sketch "Esboço30" plane through (2, 0, 0) normal (0, 0, 1) x (1, 0, 0)
  line L0 (-2, 1) -> (0, 1) projected
  line L1 (-2, 1) -> (59.7801, 1)
  line L2 (59.7801, 1) -> (59.7801, 7.8458)
  line L3 (59.7801, 7.8458) -> (-2, 7.8458)
  line L4 (-2, 7.8458) -> (-2, 1)
  point P0 (-2, 0)
  constraints: 8 end point, 2 parallel, 1 horizontal, 1 perpendicular
extrude "Extrusão26" cut sketch "Esboço30" against normal blind 500
